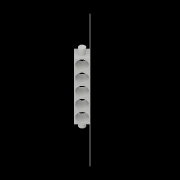
# Autodesk Inventor part: TubeHolderV2
Saved by Autodesk Inventor 2019 (Build 230136000, 136)
## iProperties
Created: 2021-09-16
Part Number: TubeHolderV2
Material: Generic
Document SubType Name: Modeling
Designer: timmy
Density: 1 g/cm^3
Appearance: Default
Author: timmy
Autodesk Inventor part; units mm, degrees
ref_plane "YZ Plane" through (0, 0, 0) normal (1, 0, 0) x (0, 1, 0)
ref_plane "Work Plane1" through (-76.2, 0, -127) normal (0.7071068, 0, -0.7071068) x (-0.7071068, 0, -0.7071068)
sketch "Sketch2" plane through (-76.2, 0, -127) normal (0.7071068, 0, -0.7071068) x (-0.7071068, 0, -0.7071068)
  line L0 (-107.7631, 0) -> (0, 0) projected
  line L1 (0, 0) -> (0, 127) projected
  line L2 (-107.7631, 127) -> (0, 127) projected
  line L3 (-107.7631, 0) -> (-107.7631, 127)
  line L4 (-107.7631, -190.5) -> (0.0091, -190.5)
  line L5 (0.0091, -190.5) -> (0.0091, 317.5)
  line L6 (0.0091, 317.5) -> (-107.7631, 317.5)
  line L7 (-107.7631, -190.5) -> (-107.7631, 317.5)
  point P0 (-143.6841, 0)
  dimension "d9" = 107.7722
  dimension "d10" = 508
  constraints: 10 end point, 2 perpendicular, 1 horizontal, 1 vertical
  measures "d9" distance of L4.start L4.end
  measures "d10" distance of L4.end L5.end
extrude "Extrusion2" add sketch "Sketch2" along normal blind 101.6
sketch "Sketch3" plane through (-76.2065, -190.5, -127.0065) normal (-0.7071068, 0, -0.7071068) x (-0.7071068, 0, 0.7071068)
  line L0 (0, 0) -> (-101.6, 0) projected
  line L1 (0, 508) -> (-101.6, 508) projected
  circle A0 centre (-50.8, 50.8) radius 44.45
  circle A1 centre (-50.8, 152.4) radius 44.45
  circle A2 centre (-50.8, 254) radius 44.45
  circle A3 centre (-50.8, 355.6) radius 44.45
  circle A4 centre (-50.8, 457.2) radius 44.45
  point P0 (35.921, 190.5)
  constraints: 5 centre point
extrude "Extrusion3" cut sketch "Sketch3" against normal blind 127
ref_plane "Work Plane2" through (-76.2065, -190.5, -127.0065) normal (0, -1, 0) x (0.7071068, 0, -0.7071068)
sketch "Sketch5" plane through (-76.2065, -190.5, -127.0065) normal (0, -1, 0) x (0.7071068, 0, -0.7071068)
  line L0 (101.6, 107.7722) -> (101.6, 0) projected
  line L1 (101.6, 53.8861) -> (0, 53.8907)
  line L2 (0, 107.7722) -> (0, 0.0091) projected
  circle A0 centre (50.8, 53.8884) radius 25.4
  point P0 (-35.921, 143.6932)
  dimension "d52" = 50.8
  constraints: 3 midpoint, 2 end point, 1 centre point
  measures "d52" diameter of A0
extrude "Extrusion5" add sketch "Sketch5" along normal blind 50.8
sketch "Sketch6" plane through (0, 317.5, -50.8) normal (0, 1, 0) x (0.7071068, 0, -0.7071068)
  line L0 (50.8, 107.779) -> (50.8, 0)
  line L1 (95.25, 0) -> (6.35, 0) projected
  circle A0 centre (50.8, 53.8895) radius 25.4
  point P0 (-35.921, -35.921)
  dimension "d55" = 50.8
  constraints: 2 end point, 2 midpoint, 1 centre point
  measures "d55" diameter of A0
extrude "Extrusion6" add sketch "Sketch6" along normal blind 50.8
sketch "Sketch7" plane through (0, -190.5, -50.8) normal (0.7071068, 0, 0.7071068) x (0.7071068, 0, -0.7071068)
  line L0 (0, 508) -> (101.6, 508) projected
  line L1 (0, 0) -> (101.6, 0) projected
  line L2 (101.6, 508) -> (100.0125, 508)
  line L3 (100.0125, 508) -> (100.0125, 0)
  line L4 (100.0125, 0) -> (101.6, 0)
  line L5 (101.6, 0) -> (101.6, 508)
  point P0 (-35.921, 190.5)
  dimension "d58" = 1.5875
  constraints: 8 end point, 2 parallel, 1 horizontal, 1 perpendicular, 1 point on line
  measures "d58" distance of L4.end L3.end
extrude "Extrusion7" add sketch "Sketch7" along normal blind 457.2
sketch "Sketch8" plane through (-76.2065, -190.5, -127.0065) normal (-0.7071068, 0, -0.7071068) x (-0.7071068, 0, 0.7071068)
  line L0 (0, 0) -> (-101.6, 0) projected
  line L1 (0, 508) -> (-101.6, 508) projected
  line L2 (-101.6, 0) -> (-100.0125, 0)
  line L3 (-100.0125, 0) -> (-100.0125, 508)
  line L4 (-100.0125, 508) -> (-101.6, 508)
  line L5 (-101.6, 508) -> (-101.6, 0)
  point P0 (35.921, 190.5)
  dimension "d61" = 1.5875
  constraints: 8 end point, 2 parallel, 1 horizontal, 1 perpendicular, 1 point on line
  measures "d61" distance of L4.end L3.end
extrude "Extrusion8" add sketch "Sketch8" along normal blind 381
sketch "Sketch9" plane through (-4.358, 0, -198.842) normal (0.7071068, 0, -0.7071068) x (-0.7071068, 0, -0.7071068)
  line L0 (-107.7631, 19.05) -> (-107.7631, 107.95) projected
  line L1 (-308.7004, -158.8821) -> (-308.7004, 285.8821) construction
  line L2 (-308.7004, 285.8821) -> (148.7714, 285.8821) construction
  line L3 (148.7714, 285.8821) -> (148.7714, -158.8821) construction
  line L4 (148.7714, -158.8821) -> (-308.7004, -158.8821) construction
  line L5 (381.0091, -190.5) -> (-564.9631, -190.5) projected
  line L6 (-564.9631, 317.5) -> (381.0091, 317.5) projected
  line L7 (-52.6357, -190.5) -> (-52.6357, -158.8821)
  line L8 (-79.2736, 317.5) -> (-28.4736, 317.5) projected
  line L9 (-52.6357, 317.5) -> (-52.6357, 285.8821)
  point P0 (-143.6841, 0)
  constraints: 6 point on line, 4 end point, 1 collinear, 1 perpendicular, 2 other
sketch "Sketch10" plane through (-4.358, 0, -198.842) normal (0.7071068, 0, -0.7071068) x (-0.7071068, 0, -0.7071068)
  arc A0 (-275.2437, 285.2481) -> (-250.9536, -157.2542) centre (270.3239, 93.2779) ccw
  line L0 (-250.9536, -157.2542) -> (-149.0408, -157.2542)
  arc A1 (-149.0408, -157.2542) -> (-3.1742, -113.4409) centre (-198.5082, 272.1584) ccw
  line L1 (-275.2437, 285.2481) -> (-178.2812, 285.2481)
  arc A2 (53.2425, 193.5012) -> (-178.2812, 285.2481) centre (-212.8493, -139.9836) ccw
  arc A3 (150.1891, 61.5781) -> (53.2425, 193.5012) centre (-192.4431, -88.6295) ccw
  arc A4 (109.0206, -17.6127) -> (150.1891, 61.5781) centre (-195.4605, 190.9724) ccw
  line L2 (109.0206, -17.6127) -> (109.0206, -41.948)
  line L3 (109.0206, -41.948) -> (98.9415, -36.1338)
  line L4 (98.9415, -36.1338) -> (98.9415, -61.6271)
  line L5 (98.9415, -61.6271) -> (90.5927, -55.3656)
  line L6 (90.5927, -55.3656) -> (90.5927, -65.6524)
  line L7 (90.5927, -65.6524) -> (86.5675, -65.6524)
  line L8 (86.5675, -65.6524) -> (75.2371, -55.3656)
  line L9 (75.2371, -55.3656) -> (60.925, -67.2923)
  line L10 (60.925, -67.2923) -> (60.925, -132.5911)
  line L11 (60.925, -132.5911) -> (53.3101, -126.8799)
  line L12 (53.3101, -126.8799) -> (53.3101, -152.7174)
  line L13 (53.3101, -152.7174) -> (44.7156, -146.2715)
  line L14 (44.7156, -146.2715) -> (44.7156, -157.2542)
  arc A5 (-3.1742, -113.4409) -> (44.7156, -157.2542) centre (94.171, -55.1178) ccw
  arc A6 (102.7461, -15.6605) -> (143.41, 61.392) centre (-195.4605, 190.9724) ccw
  arc A7 (143.41, 61.392) -> (49.2236, 188.6808) centre (-192.4431, -88.6295) ccw
  arc A8 (49.2236, 188.6808) -> (-178.5367, 278.9736) centre (-212.8493, -139.9836) ccw
  line L15 (-178.5367, 278.9736) -> (-270.7817, 278.9736)
  arc A9 (-270.7817, 278.9736) -> (-246.9926, -150.9797) centre (270.3239, 93.2779) ccw
  line L16 (-246.9926, -150.9797) -> (-149.4023, -150.9797)
  arc A10 (-149.4023, -150.9797) -> (-0.6735, -105.093) centre (-198.5082, 272.1584) ccw
  arc A11 (-0.6735, -105.093) -> (38.4411, -146.6992) centre (94.171, -55.1178) ccw
  line L17 (38.4411, -146.6992) -> (38.4411, -133.7225)
  line L18 (38.4411, -133.7225) -> (47.0356, -140.1684)
  line L19 (47.0356, -140.1684) -> (47.0356, -114.3309)
  line L20 (47.0356, -114.3309) -> (54.6505, -120.0421)
  line L21 (54.6505, -120.0421) -> (54.6505, -64.3535)
  line L22 (54.6505, -64.3535) -> (75.4135, -47.051)
  line L23 (75.4135, -47.051) -> (84.3182, -55.1356)
  line L24 (84.3182, -55.1356) -> (84.3182, -42.8166)
  line L25 (84.3182, -42.8166) -> (92.667, -49.0781)
  line L26 (92.667, -49.0781) -> (92.667, -25.2706)
  line L27 (92.667, -25.2706) -> (102.7461, -31.0849)
  line L28 (102.7461, -31.0849) -> (102.7461, -15.6605)
  line L29 (-233.3315, -107.3482) -> (-192.4431, -94.6411)
  arc A12 (-192.4431, -94.6411) -> (-194.5165, -87.9697) centre (-196.5945, -92.2734) ccw
  arc A13 (-235.2367, -100.9836) -> (-233.3315, -107.3482) centre (-234.3174, -104.1759) ccw
  line L30 (-235.2367, -100.9836) -> (-194.5165, -87.9697)
  arc A14 (-200.9643, -70.0216) -> (-204.2812, -65.6524) centre (-202.6775, -67.8785) ccw
  arc A15 (-218.593, -92.1978) -> (-212.8873, -88.6295) centre (-216.1069, -89.8273) ccw
  arc A16 (-240.0176, -97.7417) -> (-234.1801, -93.3359) centre (-236.794, -95.9427) ccw
  line L31 (-204.2812, -65.6524) -> (-218.593, -78.9038)
  line L32 (-218.593, -92.1978) -> (-221.3074, -87.3906)
  arc A17 (-218.593, -78.9038) -> (-221.3074, -87.3906) centre (-215.5705, -84.548) ccw
  line L33 (-200.9643, -70.0216) -> (-214.136, -82.5975)
  arc A18 (-214.136, -82.5975) -> (-212.8873, -88.6295) centre (-209.7391, -84.8326) ccw
  arc A19 (-249.1818, -52.8821) -> (-214.136, -41.948) centre (-232.8162, -43.7057) ccw
  arc A20 (-254.3841, -55.7023) -> (-207.5564, -41.8661) centre (-232.4405, -43.8084) ccw
  arc A21 (-249.1818, -52.8821) -> (-254.3841, -55.7023) centre (-251.9566, -53.9719) ccw
  arc A22 (-207.5564, -41.8661) -> (-214.136, -41.948) centre (-210.8436, -42.1227) ccw
  arc A23 (-257.3084, -45.9474) -> (-250.9536, -45.9474) centre (-254.131, -44.641) ccw
  arc A24 (-210.8829, -30.8723) -> (-257.3066, -36.1328) centre (-232.873, -44.2843) ccw
  arc A25 (-257.3066, -36.1328) -> (-257.3084, -45.9474) centre (-232.6841, -41.0444) ccw
  arc A26 (-216.564, -34.3315) -> (-250.9536, -45.9474) centre (-232.639, -43.4545) ccw
  arc A27 (-216.564, -34.3315) -> (-210.8829, -30.8723) centre (-213.6702, -32.6892) ccw
  arc A28 (-261.9645, -11.4459) -> (-260.3229, -17.6127) centre (-261.6163, -14.6551) ccw
  arc A29 (-222.5463, -7.0053) -> (-224.6592, -0.5544) centre (-224.214, -3.98) ccw
  arc A30 (-227.6774, 2.1966) -> (-222.3384, 1.5605) centre (-224.7247, 4.2552) ccw
  arc A31 (-266.0931, -8.0744) -> (-261.1716, -5.7425) centre (-263.6042, -6.9678) ccw
  arc A32 (-247.6785, 0.3673) -> (-244.0482, 2.2199) centre (-245.8413, 1.2503) ccw
  arc A33 (-246.5516, 14.9303) -> (-243.0661, 11.5075) centre (-244.8089, 13.2189) ccw
  arc A34 (-247.6785, 0.3673) -> (-261.1716, -5.7425) centre (-255.3014, -0.7521) ccw
  arc A35 (-227.6774, 2.1966) -> (-243.0661, 11.5075) centre (-237.254, 3.7411) ccw
  arc A36 (-222.3384, 1.5605) -> (-246.5516, 14.9303) centre (-236.224, 5.0235) ccw
  line L34 (-260.3229, -17.6127) -> (-222.5463, -7.0053)
  line L35 (-224.6592, -0.5544) -> (-261.9645, -11.4459)
  arc A37 (-244.0482, 2.2199) -> (-266.0931, -8.0744) centre (-256.3068, -0.2802) ccw
  arc A38 (-272.6937, 39.2683) -> (-278.0802, 36.6427) centre (-275.5868, 38.3654) ccw
  arc A39 (-272.6937, 39.2683) -> (-236.2212, 46.3075) centre (-255.2802, 47.0507) ccw
  arc A40 (-230.0121, 46.2453) -> (-236.2212, 46.3075) centre (-233.1175, 46.1865) ccw
  arc A41 (-278.0802, 36.6427) -> (-230.0121, 46.2453) centre (-254.9111, 45.7739) ccw
  arc A42 (-279.7753, 47.1726) -> (-274.3537, 47.049) centre (-277.0729, 46.7398) ccw
  arc A43 (-237.8071, 54.6985) -> (-274.3537, 47.049) centre (-254.9987, 45.7059) ccw
  arc A44 (-237.8071, 54.6985) -> (-232.5056, 56.6448) centre (-235.2837, 56.0185) ccw
  arc A45 (-232.5056, 56.6448) -> (-279.7753, 47.1726) centre (-255.2467, 47.4483) ccw
  line L36 (-266.0931, 110.4809) -> (-249.0901, 126.6046)
  line L37 (-266.0931, 110.4809) -> (-286.549, 125.3544)
  line L38 (-288.8332, 119.7169) -> (-270.8891, 106.3082)
  arc A46 (-286.549, 125.3544) -> (-288.8332, 119.7169) centre (-286.643, 122.111) ccw
  arc A47 (-244.0462, 121.1035) -> (-249.0901, 126.6046) centre (-246.522, 123.8964) ccw
  line L39 (-244.0462, 121.1035) -> (-262.0594, 106.2289)
  arc A48 (-270.8891, 106.3082) -> (-262.0594, 106.2289) centre (-266.4202, 112.2887) ccw
  arc A49 (-285.323, 101.2574) -> (-285.3573, 94.2931) centre (-285.3522, 97.7753) ccw
  arc A50 (-244.8089, 96.7093) -> (-244.8082, 103.6717) centre (-245.0146, 100.1905) ccw
  line L40 (-285.3573, 94.2931) -> (-244.8089, 96.7093)
  line L41 (-244.8082, 103.6717) -> (-285.323, 101.2574)
  line L42 (-287.617, 156.4561) -> (-249.1121, 135.4926)
  line L43 (-285.2431, 161.6212) -> (-245.8406, 140.6102)
  arc A51 (-249.1121, 135.4926) -> (-245.8406, 140.6102) centre (-247.6564, 138.1665) ccw
  arc A52 (-285.2431, 161.6212) -> (-287.617, 156.4561) centre (-286.5828, 159.1089) ccw
  line L44 (-257.7917, 164.633) -> (-273.3535, 158.7092)
  line L45 (-257.7917, 164.633) -> (-257.7917, 150.5688)
  arc A53 (-257.7917, 150.5688) -> (-250.9536, 150.5688) centre (-254.3727, 152.2296) ccw
  line L46 (-250.9536, 166.6462) -> (-250.9536, 150.5688)
  line L47 (-250.9536, 166.6462) -> (-242.0329, 169.9488)
  arc A54 (-242.0329, 169.9488) -> (-244.0462, 175.3869) centre (-243.5166, 172.4912) ccw
  arc A55 (-275.2437, 165.111) -> (-273.3535, 158.7092) centre (-273.7037, 162.0857) ccw
  line L48 (-275.2437, 165.111) -> (-244.0462, 175.3869)
  line L49 (-279.2889, 186.5617) -> (-272.3261, 211.4267)
  line L50 (-285.2491, 189.9216) -> (-278.5099, 213.988)
  arc A56 (-285.2491, 189.9216) -> (-279.2889, 186.5617) centre (-281.8574, 188.9719) ccw
  arc A57 (-272.3261, 211.4267) -> (-278.5099, 213.988) centre (-275.4547, 212.6188) ccw
  line L51 (-270.7822, 195.4202) -> (-242.0071, 186.5537)
  arc A58 (-242.0071, 186.5537) -> (-239.2233, 193.8829) centre (-240.8504, 190.3077) ccw
  arc A59 (-269.3808, 201.9548) -> (-270.7822, 195.4202) centre (-269.7944, 198.6259) ccw
  line L52 (-269.3808, 201.9548) -> (-239.2233, 193.8829)
  line L53 (-265.5726, 228.372) -> (-258.8339, 241.1013)
  line L54 (-270.2745, 232.5331) -> (-265.0656, 244.0628)
  arc A60 (-270.2745, 232.5331) -> (-265.5726, 228.372) centre (-267.719, 230.6837) ccw
  arc A61 (-258.8339, 241.1013) -> (-265.0656, 244.0628) centre (-261.8857, 242.7169) ccw
  line L55 (-258.9463, 249.6693) -> (-234.1801, 210.6089)
  arc A62 (-234.1801, 210.6089) -> (-229.2768, 214.0214) centre (-231.6551, 212.2098) ccw
  arc A63 (-254.138, 253.374) -> (-258.9463, 249.6693) centre (-256.3724, 251.3013) ccw
  line L56 (-229.2768, 214.0214) -> (-254.138, 253.374)
  arc A64 (-229.2768, 222.6474) -> (-224.6592, 218.8667) centre (-227.0075, 220.7089) ccw
  line L57 (-229.2768, 222.6474) -> (-223.3293, 233.2803)
  line L58 (-224.6592, 218.8667) -> (-217.4787, 231.3142)
  arc A65 (-217.4787, 231.3142) -> (-223.3293, 233.2803) centre (-220.5364, 231.9033) ccw
  line L59 (-240.0176, -97.7417) -> (-242.5425, -90.8551)
  arc A66 (-223.3293, -72.9688) -> (-242.5425, -90.8551) centre (-228.8554, -86.2952) ccw
  arc A67 (-224.6592, -79.8539) -> (-223.3293, -72.9688) centre (-224.0401, -76.4025) ccw
  arc A68 (-224.6592, -79.8539) -> (-234.1801, -93.3359) centre (-227.0878, -88.2416) ccw
  point P0 (-143.6841, 0)
  constraints: 143 point on circle, 120 end point, 69 centre point, 16 tangent, 15 parallel, 3 vertical, 2 horizontal, 1 perpendicular, 17 other
extrude "Extrusion10" cut sketch "Sketch10" against normal up to surface (1.5875 mm away) contours L1 A2 A3 A4 L2 L3 L4 L5 L6 L7 L8 L9 L10 L11 L12 L13 L14 A5 A1 L0 A0 | A13 L30 A12 L29 | L33 A18 A15 L32 A17 L31 A14 | A19 A22 A20 A21 | A25 A24 A27 A26 A23 | L35 A29 L34 A28 | A35 A33 A36 A30 | A37 A32 A34 A31 | A39 A40 A41 A38 | A45 A44 A43 A42 | L36 A47 L39 A48 L38 A46 L37 | L41 A50 L40 A49 | A52 L43 A51 L42 | L44 A55 L48 A54 L47 L46 A53 L45 | A56 L50 A57 L49 | A59 L52 A58 L51 | A60 L54 A61 L53 | A63 L56 A62 L55 | L57 A65 L58 A64
body "Solid1"
